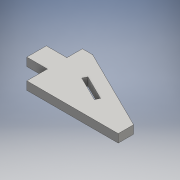
# Autodesk Inventor part: display support
Saved by Autodesk Inventor 2016 SP1 (Build 200210100, 210)
## iProperties
Created: 2016-04-07
Part Number: display support
Material: Generic
Document SubType Name: Modeling
Designer: ubik
Density: 1 g/cm^3
Appearance: Default
Author: ubik
Autodesk Inventor part; units mm, degrees
ref_plane "YZ Plane" through (0, 0, 0) normal (1, 0, 0) x (0, 1, 0)
ref_plane "XZ Plane" through (0, 0, 0) normal (0, 1, 0) x (-1, 0, 0)
ref_plane "XY Plane" through (0, 0, 0) normal (0, 0, 1) x (1, 0, 0)
sketch "Sketch1" plane through (0, 0, 0) normal (0, 0, 1) x (1, 0, 0)
  line L0 (-10, 9.5) -> (10, 9.5)
  line L1 (10, 9.5) -> (10, -9.5)
  line L2 (10, -9.5) -> (-10, -9.5)
  line L3 (-10, -9.5) -> (-10, 9.5)
  line L4 (10, 9.5) -> (10, 24.5)
  line L5 (10, 24.5) -> (20, 24.5)
  line L6 (20, 24.5) -> (98.8731, -14.5261)
  line L7 (98.8731, -14.5261) -> (98.8731, -24.5261)
  line L8 (10, -9.5) -> (10, -29.5)
  line L9 (10, -29.5) -> (98.8731, -29.5)
  line L10 (98.8731, -29.5) -> (98.8731, -24.5261)
  point P0 (0, 0)
  dimension "d0" = 20
  dimension "d1" = 19
  dimension "d2" = 9.5
  dimension "d3" = 10
  dimension "d4" = 15
  dimension "d5" = 10
  dimension "d6" = 10
  dimension "d7" = 88
  dimension "d8" = 20
  constraints: 22 end point, 4 perpendicular, 3 parallel, 2 vertical, 1 horizontal, 1 point on line
  measures "d0" distance of L0.start L0.end
  measures "d1" distance of L2.end L0.start
  measures "d2" distance from line of point (0, 0) L0
  measures "d3" distance from line of point (0, 0) L3
  measures "d4" distance of L0.end L4.end
  measures "d5" distance of L4.end L5.end
  measures "d6" distance of L6.end L7.end
  measures "d7" distance of L5.end L6.end
  measures "d8" distance of L1.end L8.end
extrude "Extrusion1" add sketch "Sketch1" along normal blind 8
sketch "Sketch2" plane through (0, 0, 8) normal (0, 0, 1) x (1, 0, 0)
  line L0 (98.8731, -14.5261) -> (20, 24.5) projected
  line L1 (41.5108, 13.8565) -> (34.4152, -0.484)
  line L2 (34.4152, -0.484) -> (58.6149, -12.4579)
  line L3 (58.6149, -12.4579) -> (65.7105, 1.8826)
  line L4 (36.4108, 3.5492) -> (60.6106, -8.4247)
  point P0 (0, 0)
  dimension "d12" = 24
  dimension "d13" = 27
  dimension "d17" = 16
  dimension "d18" = 4.5
  constraints: 8 end point, 4 perpendicular, 4 point on line
  measures "d12" distance from line of L0.end L1
  measures "d13" distance of L1.end L2.end
  measures "d17" distance between parallel lines of L0 L2
  measures "d18" distance between parallel lines of L2 L4
extrude "Extrusion3" cut sketch "Sketch2" against normal through all contours L3 L2 L1 L4
equation "\"d2\" = 0.5 * d1"
equation "\"d3\" = 0.5 * d0"
body "Solid1"
